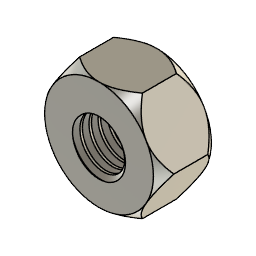
Nut_ (Autodesk Fusion 360 design; units mm, degrees)
Autodesk Fusion 360 part; units mm, degrees
sketch "Sketch1" plane through (0, 0, 0) normal (0, 1, 0) x (1, 0, 0)
  circle A0 centre (0, 0) radius 4
  line L0 (4.3301, -7.5) -> (8.6603, 0)
  line L1 (8.6603, 0) -> (4.3301, 7.5)
  line L2 (4.3301, 7.5) -> (-4.3301, 7.5)
  line L3 (-4.3301, 7.5) -> (-8.6603, 0)
  line L4 (-8.6603, 0) -> (-4.3301, -7.5)
  line L5 (-4.3301, -7.5) -> (4.3301, -7.5)
  dimension "d1" = 8
  dimension "d2" = 15
  constraint coincident A0.centre origin
  constraint horizontal L3.end A0.centre
  measures "d1" diameter of A0
  measures "d2" distance of L2 L5
extrude "Extrude1" add sketch "Sketch1" along normal mid plane 8
sketch "Sketch2" plane through (0, -4, 0) normal (0, -1, 0) x (1, 0, 0)
  circle A0 centre (0, 0) radius 4
  line L0 (4.3301, 7.5) -> (-4.3301, 7.5)
  line L1 (-4.3301, 7.5) -> (-8.6603, 0)
  line L2 (-8.6603, 0) -> (-4.3301, -7.5)
  line L3 (-4.3301, -7.5) -> (4.3301, -7.5)
  line L4 (4.3301, -7.5) -> (8.6603, 0)
  line L5 (8.6603, 0) -> (4.3301, 7.5)
  circle A1 centre (0, 0) radius 7.5
  dimension "d5" = 15
  constraint coincident A0.centre A1.centre
  measures "d5" diameter of A1
extrude "Extrude2" cut sketch "Sketch2" against normal through all draft 35 contours A1 keep common part
mirror "Mirror1" about plane through (0, 0, 0) normal (0, 1, 0) of "Extrude2"
thread "Thread1" "ISO Metric profile 8.0 M8x1.25 M8x1.25 6H" major diameter 8.17 minor diameter 6.7795 pitch 1.25 angle 60 modelled right hand crest width 0.343 on face at (3.995, 1.3333, 0.1994) crest through (3.3898, -3.6875, 0)
